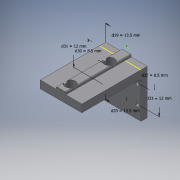
# Autodesk Inventor part: CameraMountA
Saved by Autodesk Inventor 2018.2 (Build 222227000, 227)
## iProperties
Created: 2019-05-07
Part Number: CameraMountA
Material: Generic
Vendor: HHMI: JRC - ID&F
Document SubType Name: Modeling
Designer: sawtelles
Density: 1 g/cm^3
Appearance: Default
RuleStatus: InUse
AfterDocSave0: file://Part Number Cleaner
DESIGN DEPARTMENT: HHMI: JRC - ID&F
ALTERED ITEM PART NUMBER: N/A
ALTERED ITEM VENDOR: N/A
ALTERED ITEM DESCRIPTION: N/A
Author: sawtelles
Revision Number: 0
Autodesk Inventor part; units mm, degrees
ref_plane "YZ Plane" through (0, 0, 0) normal (1, 0, 0) x (0, 1, 0)
ref_plane "XZ Plane" through (0, 0, 0) normal (0, 1, 0) x (-1, 0, 0)
ref_plane "XY Plane" through (0, 0, 0) normal (0, 0, 1) x (1, 0, 0)
sketch "Sketch1" plane through (0, 0, 0) normal (0, 0, 1) x (1, 0, 0)
  line L0 (0, 0) -> (27, 0)
  line L1 (27, 0) -> (27, 29)
  line L2 (27, 29) -> (0, 29)
  line L3 (0, 29) -> (0, 0)
  dimension "d0" = 27
  dimension "d1" = 29
  constraints: 8 end point, 2 parallel, 1 horizontal, 1 perpendicular
  measures "d0" distance of L2.end L1.end
  measures "d1" distance of L1.end L0.end
extrude "Extrusion1" add sketch "Sketch1" along normal blind 4
sketch "Sketch2" plane through (0, 0, 4) normal (0, 0, 1) x (1, 0, 0)
  line L0 (27, 29) -> (0, 29) projected
  point P0 (0, 0)
  point P1 (2.5, 20.5)
  point P2 (24.5, 20.5)
  point P3 (2.5, 8.5)
  point P4 (24.5, 8.5)
  dimension "d30" = 8.5
  dimension "d31" = 12
  dimension "d32" = 8.5
  dimension "d33" = 12
  measures "d30" distance from line of L0 point (2.5, 20.5)
  measures "d31" distance of point (2.5, 20.5) point (2.5, 8.5)
  measures "d32" distance from line of L0 point (24.5, 20.5)
  measures "d33" distance of point (24.5, 20.5) point (24.5, 8.5)
sketch "Sketch3" plane through (0, 0, 0) normal (0, 0, -1) x (-1, 0, 0)
  line L0 (0, 29) -> (0, 0) projected
  point P0 (-13.5, 33)
  point P1 (-13.5, 5)
  dimension "d19" = 13.5
  dimension "d20" = 13.5
  measures "d19" distance from line of point (-13.5, 33) L0
  measures "d20" distance from line of point (-13.5, 5) L0
sketch "Sketch6" plane through (0, 0, 4) normal (0, 0, 1) x (1, 0, 0)
  line L0 (0, 29) -> (0, 0) projected
  line L1 (27, 0) -> (27, 29) projected
  line L2 (0, 29) -> (27, 29)
  line L3 (27, 29) -> (27, 24)
  line L4 (27, 24) -> (0, 24)
  line L5 (0, 24) -> (0, 29)
  dimension "d34" = 5
  constraints: 8 end point, 2 parallel, 1 horizontal, 1 perpendicular, 1 point on line
  measures "d34" distance of L2.end L3.end
extrude "Extrusion4" add sketch "Sketch6" along normal blind 38.4
sketch "Sketch8" plane through (0, 29, 0) normal (0, 1, 0) x (1, 0, 0)
  line L0 (0, 0) -> (27, 0) projected
  line L1 (0, -42.4) -> (27, -42.4) projected
  line L2 (10.35, 0) -> (16.65, 0)
  line L3 (16.65, 0) -> (16.65, -42.4)
  line L4 (16.65, -42.4) -> (10.35, -42.4)
  line L5 (10.35, -42.4) -> (10.35, 0)
  line L6 (0, 0) -> (0, -42.4) projected
  dimension "d41" = 6.3
  dimension "d51" = 10.35
  constraints: 8 end point, 2 parallel, 2 point on line, 1 horizontal, 1 perpendicular
  measures "d41" distance of L3.end L4.end
  measures "d51" distance between parallel lines of L5 L6
extrude "Extrusion6" add sketch "Sketch8" along normal blind 1.5 contours L0 L3 L1 L5
sketch "Sketch9" plane through (0, 24, 4) normal (0, -1, 0) x (1, 0, 0)
  line L0 (0, 0) -> (27, 0) projected
  point P0 (0, -4)
  point P1 (13.5, 7)
  point P2 (13.5, 20)
  dimension "d69" = 7
  measures "d69" distance from line of L0 point (13.5, 7)
hole "Hole3" at (13.5, 24, 11) direction (0, 1, 0) diameter 6.6 end through all
fillet "Fillet1" radius 2 1 edges at (13.5, 24, 4)
sketch "Sketch10" plane through (0, 0, 4) normal (0, 0, 1) x (1, 0, 0)
  line L0 (24.5, 20.9) -> (24.5, 20.1) construction
  line L1 (23.4, 20.9) -> (23.4, 20.1)
  line L2 (25.6, 20.1) -> (25.6, 20.9)
  arc A0 (25.6, 20.9) -> (23.4, 20.9) centre (24.5, 20.9) ccw
  arc A1 (23.4, 20.1) -> (25.6, 20.1) centre (24.5, 20.1) ccw
  line L3 (24.5, 8.9) -> (24.5, 8.1) construction
  line L4 (23.4, 8.9) -> (23.4, 8.1)
  line L5 (25.6, 8.1) -> (25.6, 8.9)
  arc A2 (25.6, 8.9) -> (23.4, 8.9) centre (24.5, 8.9) ccw
  arc A3 (23.4, 8.1) -> (25.6, 8.1) centre (24.5, 8.1) ccw
  line L6 (2.5, 20.9) -> (2.5, 20.1) construction
  line L7 (1.4, 20.9) -> (1.4, 20.1)
  line L8 (3.6, 20.1) -> (3.6, 20.9)
  arc A4 (3.6, 20.9) -> (1.4, 20.9) centre (2.5, 20.9) ccw
  arc A5 (1.4, 20.1) -> (3.6, 20.1) centre (2.5, 20.1) ccw
  line L9 (2.5, 8.1) -> (2.5, 8.9) construction
  line L10 (3.6, 8.1) -> (3.6, 8.9)
  line L11 (1.4, 8.9) -> (1.4, 8.1)
  arc A6 (1.4, 8.1) -> (3.6, 8.1) centre (2.5, 8.1) ccw
  arc A7 (3.6, 8.9) -> (1.4, 8.9) centre (2.5, 8.9) ccw
  point P0 (0, 0)
  point P1 (24.5, 20.5)
  point P2 (24.5, 8.5)
  point P3 (2.5, 20.5)
  point P4 (2.5, 8.5)
  dimension "d53" = 0.4
  dimension "d54" = 2.2
  dimension "d55" = 0.4
  dimension "d56" = 2.2
  dimension "d57" = 0.4
  dimension "d58" = 2.2
  dimension "d59" = 0.4
  dimension "d60" = 2.2
  constraints: 32 end point, 16 point on circle, 16 tangent, 8 centre point, 5 parallel, 4 midpoint, 3 vertical
  measures "d53" distance of point (24.5, 20.5) L0.end
  measures "d54" diameter of A1
  measures "d55" distance of point (24.5, 8.5) L3.end
  measures "d56" diameter of A3
  measures "d57" distance of point (2.5, 20.5) L6.end
  measures "d58" diameter of A5
  measures "d59" distance of point (2.5, 8.5) L9.end
  measures "d60" diameter of A7
extrude "Extrusion7" cut sketch "Sketch10" against normal through all
chamfer "Chamfer1" distance 0.4 angle 45 1 edges at (16.65, 30.5, 27.1918)
chamfer "Chamfer2" distance 0.4 angle 45 3 edges at (16.65, 30.5, 5.0082) (10.35, 30.5, 27.1918) (10.35, 30.5, 5.0082)
sketch "Sketch11" plane through (0, 24, 42.4) normal (0, -1, 0) x (1, 0, 0)
  point P0 (0, -42.4)
  point P1 (13.5, -6)
hole "Hole4" at (13.5, 24, 36.4) direction (0, 1, 0) diameter 6.6 end through all
body "Solid1"
